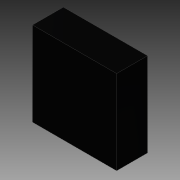
# Autodesk Inventor part: XFL3010
Saved by Autodesk Inventor 2013 (Build 170138000, 138)
## iProperties
Created: 2015-07-04
Part Number: XFL3010
Material: Ogólny
Document SubType Name: Modeling
Designer: terg
Density: 1 g/cm^3
Author: terg
Autodesk Inventor part; units mm, degrees
ref_plane "YZ Plane" through (0, 0, 0) normal (1, 0, 0) x (0, 1, 0)
ref_plane "XZ Plane" through (0, 0, 0) normal (0, 1, 0) x (-1, 0, 0)
ref_plane "XY Plane" through (0, 0, 0) normal (0, 0, 1) x (1, 0, 0)
sketch "Szkic1" plane through (0, 0, 0) normal (0, 1, 0) x (-1, 0, 0)
  line L0 (0, 0) -> (-3, 0)
  line L1 (-3, 0) -> (-3, -3)
  line L2 (-3, -3) -> (0, -3)
  line L3 (0, -3) -> (0, 0)
  dimension "d0" = 3
  dimension "d1" = 3
  constraints: 8 end point, 2 parallel, 1 horizontal, 1 perpendicular
  measures "d0" distance of L2.end L1.end
  measures "d1" distance of L1.end L0.end
extrude "Wyciągnięcie proste1" add sketch "Szkic1" along normal blind 1.1
sketch "Szkic2" plane through (0, 1.1, 0) normal (0, 1, 0) x (1, 0, 0)
  line L0 (0, 3) -> (0, 0) projected
  spline S0 degree 4 poles (1.6944, 2.1983) (1.9716, 2.511) (1.4563, 2.727) (0.465, 2.1643) (1.5453, 1.3461) (1.9081, 1.8041) knots 0 0 0 0 0 0.450582 1 1 1 1 1
  spline S1 degree 4 poles (1.7996, 2.1884) (2.0597, 2.5341) (1.506, 3.0725) (0.1344, 1.9443) (1.5513, 1.2446) (1.9975, 1.7232) knots 0 0 0 0 0 0.451956 1 1 1 1 1
  line L1 (1.6944, 2.1983) -> (1.8069, 2.1983)
  line L2 (1.9081, 1.8041) -> (1.9975, 1.7232)
  line L3 (0.8383, 1.1084) -> (0.9683, 1.1084)
  line L4 (0.9683, 1.1084) -> (0.9683, 0.4084)
  line L5 (0.9683, 0.4084) -> (0.8383, 0.4084)
  line L6 (0.8383, 0.4084) -> (0.8383, 1.1084)
  line L7 (0.5968, 0.8566) -> (0.7468, 0.8566)
  line L8 (0.5968, 0.8566) -> (0.8383, 1.1084)
  line L9 (0.7468, 0.8566) -> (0.8383, 0.9385)
  ellipse E0 centre (1.4307, 0.7584) end of major axis (1.4307, 0.4084) minor radius 0.2548
  ellipse E1 centre (1.4307, 0.7584) end of major axis (1.4307, 0.5022) minor radius 0.161
  arc A0 (2.2664, 0.8011) -> (1.8927, 0.8794) centre (2.0918, 0.8986) ccw
  arc A1 (2.17, 0.8011) -> (1.9683, 0.8794) centre (2.0918, 0.8986) ccw
  line L10 (1.8927, 0.8794) -> (1.9683, 0.8794)
  line L11 (2.17, 0.8011) -> (2.2664, 0.8011)
  line L12 (1.8869, 0.4884) -> (2.3869, 0.4884)
  line L13 (2.3869, 0.4884) -> (2.3869, 0.4084)
  line L14 (2.3869, 0.4084) -> (1.8869, 0.4084)
  line L15 (1.8869, 0.4084) -> (1.8869, 0.4884)
  line L16 (2.17, 0.8011) -> (1.8869, 0.4884)
  line L17 (2.2664, 0.8011) -> (2.042, 0.4884)
  point P0 (1.4399, 2.5011)
  point P1 (1.1013, 2.2094)
  point P2 (1.2284, 1.7658)
  point P3 (1.7651, 2.4967)
  point P4 (1.8334, 2.577)
  point P5 (1.435, 2.6153)
  point P6 (0.9802, 2.1884)
  point P7 (1.1387, 1.6641)
  dimension "d8" = 0.13
  dimension "d9" = 0.7
  dimension "d10" = 0.15
  dimension "d11" = 0.35
  dimension "d12" = 0.4
  dimension "d13" = 0.25
  dimension "d14" = 0.5
  dimension "d15" = 0.08
  dimension "d16" = 0.35
  dimension "d19" = 0.4625
  dimension "d20" = 0.462
  constraints: 34 end point, 5 parallel, 5 perpendicular, 4 point on circle, 3 horizontal, 2 centre point, 2 coincident, 2 point on line, 1 vertical, 17 other
  measures "d8" distance of L4.end L5.end
  measures "d9" distance of L3.end L4.end
  measures "d10" distance of L7.start L7.end
  measures "d11" distance from line of point (1.431, 0.758) L3
  measures "d12" diameter of A0
  measures "d13" diameter of A1
  measures "d14" distance of L13.end L14.end
  measures "d15" distance of L12.end L13.end
  measures "d16" distance from line of point (1.431, 0.758) L14
  measures "d19" distance from line of L4 point (1.431, 0.758)
  measures "d20" horizontal distance of point (1.431, 0.758) L10.start
extrude "Wyciągnięcie proste2" cut sketch "Szkic2" against normal blind 0.1
